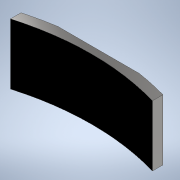
# Autodesk Inventor part: TV
Saved by Autodesk Inventor 2022 (Build 260153000, 153)
## iProperties
Created: 2022-05-13
Part Number: TV
Material: Generic
Document SubType Name: Modeling
Designer: mihir
Density: 1 g/cm^3
Appearance: Default
Author: mihir
Autodesk Inventor part; units mm, degrees
ref_plane "YZ Plane" through (0, 0, 0) normal (1, 0, 0) x (0, 1, 0)
ref_plane "XZ Plane" through (0, 0, 0) normal (0, 1, 0) x (-1, 0, 0)
ref_plane "XY Plane" through (0, 0, 0) normal (0, 0, 1) x (1, 0, 0)
sketch "Sketch1" plane through (0, 0, 0) normal (0, 1, 0) x (-1, 0, 0)
  arc A0 (0, 65.2105) -> (70, 65.2105) centre (35, 185.2105) ccw
  line L0 (70, 65.2105) -> (70, 60.0107)
  line L1 (0, 65.2105) -> (0, 60.0107)
  line L2 (15, 56.7582) -> (55, 56.7582)
  arc A1 (0, 60.0107) -> (15, 56.7582) centre (35, 185.2105) ccw
  arc A2 (55, 56.7582) -> (70, 60.0107) centre (35, 185.2105) ccw
  point P0 (0, 0)
  point P1 (35, 60.2105)
  dimension "d0" = 70
  dimension "d1" = 35
  dimension "d2" = 5
  dimension "d4" = 40
  constraints: 7 point on circle, 6 end point, 3 centre point, 1 horizontal, 1 parallel, 1 vertical
  measures "d0" distance of L1.start L0.start
  measures "d1" horizontal distance of point (35, 60.211) L1.start
  measures "d2" vertical distance of L1.start point (35, 60.211)
  measures "d4" distance of L2.start L2.end
extrude "Extrusion1" add sketch "Sketch1" along normal blind 30
body "Solid1"
